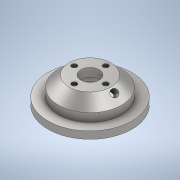
# Autodesk Inventor part: Part1
Saved by Autodesk Inventor 2021 (Build 250183000, 183)
## iProperties
Created: 2022-08-15
Part Number: Part1
Material: Stainless Steel
Document SubType Name: Sheet Metal
Designer: pc
Density: 8 g/cm^3
Sheet Metal Rule: Default_mm
Appearance: Stainless - Brushed
Mass: 3185.1 g
Surface Area: 658.474 cm^2
Volume: 398.137 cm^3
Author: pc
Autodesk Inventor part; units mm, degrees
ref_plane "XZ Plane" through (0, 0, 0) normal (0, 1, 0) x (-1, 0, 0)
ref_plane "XY Plane" through (0, 0, 0) normal (0, 0, 1) x (1, 0, 0)
sketch "Sketch1" plane through (0, 0, 0) normal (0, 0, 1) x (1, 0, 0)
  line L0 (0, 0) -> (0, 66)
  line L1 (80, 0) -> (80, 13.8071)
  line L2 (-21.5975, 0) -> (0, 0)
  line L3 (46.9201, 0) -> (53.1744, 0)
  line L4 (80, 13.8071) -> (60, 13.8071)
  line L5 (60, 13.8071) -> (60, 33.8071)
  line L6 (36.9201, 33.8071) -> (30.3778, 33.8071)
  line L7 (0, 33.8071) -> (31.3863, 33.8071)
  line L8 (0, 33.8071) -> (0, 49.8071)
  line L9 (0, 49.8071) -> (35, 49.8071)
  line L10 (46.9201, 9.2823) -> (41.9201, 9.2823)
  line L11 (41.9201, 9.2823) -> (41.9201, 33.8071)
  line L12 (41.9201, 33.8071) -> (36.9201, 33.8071)
  line L13 (60, 33.8071) -> (60, 49.8071)
  line L14 (60, 49.8071) -> (35, 49.8071)
  line L15 (46.9201, 9.2823) -> (50, 9.2823)
  line L16 (50, 9.2823) -> (50, 0)
  line L17 (50, 0) -> (80, 0)
  dimension "d0" = 66
  dimension "d2" = 160
  dimension "d4" = 20
  dimension "d5" = 20
  dimension "d15" = 35
  dimension "d16" = 70
  dimension "d84" = 100
  constraints: 36 end point, 6 horizontal, 6 perpendicular, 4 vertical, 1 point on line
  measures "d0" distance of L0.start L0.end
  measures "d2" diameter of L1 L0
  measures "d4" distance of L1.end L4.end
  measures "d5" distance of L4.end L5.end
  measures "d15" distance of L8.end L9.end
  measures "d16" diameter of L9.end L0
  measures "d84" diameter of L16 L0
revolve "Revolution1" add sketch "Sketch1" angle 360 about axis through (0, 0, 0) along (0, 1, 0)
chamfer "Chamfer1" distance 20 angle 45 1 edges at (-60, 49.8071, 0)
ref_plane "Work Plane1" through (60, 0, 0) normal (1, 0, 0) x (0, 1, 0)
sketch "Sketch8" plane through (60, 0, 0) normal (1, 0, 0) x (0, 1, 0)
  circle A0 centre (51.2317, 0) radius 7.5
  point P0 (0, 0)
  dimension "d51" = 15
  constraints: 1 centre point
  measures "d51" diameter of A0
sketch "Sketch9" plane through (0, 0, 0) normal (0, 0, 1) x (1, 0, 0)
  line L0 (60.0797, 51.2451) -> (19.226, 26.5879)
  point P0 (0, 0)
  constraints: 2 end point
sweep "Sweep2" cut profiles "Sketch8" path "Sketch9"
sketch "Sketch10" plane through (0, 49.8071, 0) normal (0, 1, 0) x (1, 0, 0)
  circle A0 centre (0, 0) radius 16
  dimension "d54" = 32
  constraints: 1 centre point, 1 coincident
  measures "d54" diameter of A0
hole "Hole2" at (0, 49.8071, 0) direction (0, -1, 0) diameter 35 end through all
sketch "Sketch11" plane through (0, 49.8071, 0) normal (0, 1, 0) x (1, 0, 0)
  circle A0 centre (0, 0) radius 40
  circle A1 centre (0, -30) radius 5
  circle A2 centre (30, 0) radius 5
  circle A3 centre (0, 30) radius 5
  circle A4 centre (-30, 0) radius 5
  dimension "d64" = 80
  dimension "d65" = 10
  dimension "d66" = 30
  dimension "d67" = 360
  constraints: 5 centre point, 1 coincident, 9 other
  measures "d64" diameter of A0
  measures "d65" diameter of A1
  measures "d66" distance of A1.centre point (0, 0)
hole "Hole3" at (0, 49.8071, -30) at (30, 49.8071, 0) at (0, 49.8071, 30) at (-30, 49.8071, 0) direction (0, -1, 0) diameter 10 depth 5 tip angle 118
thread "Thread5"
thread "Thread6"
thread "Thread7"
thread "Thread8"
equation "\"d60\" = Thickness"
equation "\"BendRadius\" = Thickness"
equation "\"BendReliefWidth\" = Thickness"
equation "\"BendReliefDepth\" = 0.5 * Thickness"
equation "\"CornerReliefSize\" = 4 * Thickness"
equation "\"MinimumRemnant\" = 2 * Thickness"
equation "\"TransitionRadius\" = BendRadius"
equation "\"JacobiRadiusSize\" = BendRadius"
equation "\"GapSize\" = Thickness"
equation "\"Thickness\" = 0.5"
body "Solid1"
